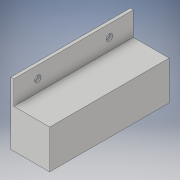
# Autodesk Inventor part: electricalCover
Saved by Autodesk Inventor 2017 SP1 (Build 210196100, 196)
## iProperties
Created: 2016-10-03
Part Number: electricalCover
Material: Generic
Document SubType Name: Modeling
Designer: steele
Density: 1 g/cm^3
Appearance: Default
Author: steele
Autodesk Inventor part; units mm, degrees
ref_plane "YZ Plane" through (0, 0, 0) normal (1, 0, 0) x (0, 1, 0)
ref_plane "XZ Plane" through (0, 0, 0) normal (0, 1, 0) x (-1, 0, 0)
ref_plane "XY Plane" through (0, 0, 0) normal (0, 0, 1) x (1, 0, 0)
sketch "Sketch1" plane through (0, 0, 0) normal (0, 0, 1) x (1, 0, 0)
  line L0 (0, 66.675) -> (0, 38.1)
  line L1 (0, 66.675) -> (3.175, 66.675)
  line L2 (3.175, 66.675) -> (3.175, 41.275)
  line L3 (3.175, 41.275) -> (41.275, 41.275)
  line L4 (41.275, 41.275) -> (41.275, 0)
  line L5 (41.275, 0) -> (38.1, 0)
  line L6 (38.1, 0) -> (38.1, 38.1)
  line L7 (38.1, 38.1) -> (0, 38.1)
  point P0 (0, 0)
  dimension "d0" = 3.175
  dimension "d1" = 3.175
  dimension "d2" = 3.175
  dimension "d3" = 38.1
  dimension "d4" = 38.1
  dimension "d5" = 25.4
  constraints: 16 end point, 5 perpendicular, 2 vertical, 1 horizontal
  measures "d0" distance of L4.end L5.end
  measures "d1" distance between parallel lines of L7 L3
  measures "d2" distance of L0.start L1.end
  measures "d3" distance from line of L6 point (0, 0)
  measures "d4" distance from line of L7 point (0, 0)
  measures "d5" distance from line of L1.end L3
extrude "Extrusion1" add sketch "Sketch1" along normal mid plane 127
sketch "Sketch2" plane through (0, 0, 63.5) normal (0, 0, 1) x (1, 0, 0)
  line L0 (0, 38.1) -> (38.1, 38.1) projected
  line L1 (38.1, 38.1) -> (38.1, 0) projected
  line L2 (0, 38.1) -> (38.1, 38.1)
  line L3 (38.1, 38.1) -> (38.1, 0)
  line L4 (38.1, 0) -> (0, 0)
  line L5 (0, 0) -> (0, 38.1)
  point P0 (0, 0)
  constraints: 8 end point, 2 parallel, 1 horizontal, 1 perpendicular
extrude "Extrusion2" add sketch "Sketch2" against normal blind 3.175
sketch "Sketch3" plane through (0, 0, -63.5) normal (0, 0, -1) x (-1, 0, 0)
  line L0 (-38.1, 38.1) -> (0, 38.1) projected
  line L1 (0, 0) -> (0, 38.1) projected
  line L2 (-38.1, 38.1) -> (0, 38.1)
  line L3 (0, 38.1) -> (0, 0)
  line L4 (0, 0) -> (-38.1, 0)
  line L5 (-38.1, 0) -> (-38.1, 38.1)
  constraints: 8 end point, 2 parallel, 1 horizontal, 1 perpendicular
extrude "Extrusion3" add sketch "Sketch3" against normal blind 3.175
sketch "Sketch4" plane through (3.175, 41.275, 63.5) normal (1, 0, 0) x (0, 0, -1)
  line L0 (0, 0) -> (0, 25.4) construction
  line L1 (0, 12.7) -> (127, 12.7) construction
  line L2 (127, 25.4) -> (127, 0) construction
  point P0 (63.5, -41.275)
  point P1 (25.4, 12.7)
  point P2 (101.6, 12.7)
  dimension "d12" = 76.2
  dimension "d13" = 25.4
  constraints: 2 end point, 2 midpoint, 2 point on line
  measures "d12" distance of point (101.6, 12.7) point (25.4, 12.7)
  measures "d13" distance of point (25.4, 12.7) L1.start
hole "Hole1" at (3.175, 53.975, 38.1) at (3.175, 53.975, -38.1) direction (-1, 0, 0) diameter 6.7564 end through all clearance for "Flat Head Machine Screw (82)" size "1/4" standard "Ansi Unified Screw Threads"
equation "\"d0\" = materialWidth"
equation "\"d1\" = materialWidth"
equation "\"d2\" = materialWidth"
equation "\"d3\" = plugDepth"
equation "\"d4\" = plugHeight"
equation "\"d5\" = heightForBolts"
equation "\"d6\" = overallWidth"
equation "\"d8\" = materialWidth"
equation "\"d10\" = materialWidth"
equation "\"d12\" = distanceBetweenBolts"
equation "\"d13\" = distanceEdgeToBoltHoles"
equation "\"overallWidth\" = 127"
equation "\"extendFromWall\" = 63.5"
equation "\"heightForBolts\" = 25.4"
equation "\"materialWidth\" = 3.175"
equation "\"plugHeight\" = 38.1"
equation "\"plugDepth\" = 38.1"
equation "\"distanceBetweenBolts\" = overallWidth - 2 * distanceEdgeToBoltHoles"
equation "\"distanceEdgeToBoltHoles\" = 25.4"
body "Solid1"
